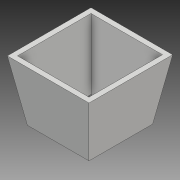
# Autodesk Inventor part: Antenna
Saved by Autodesk Inventor 2017 (Build 210142000, 142)
## iProperties
Created: 2017-01-02
Part Number: Antenna
Material: Generic
Document SubType Name: Modeling
Designer: Sachin Konan
Density: 1 g/cm^3
Appearance: Default
Author: Sachin Konan
Autodesk Inventor part; units mm, degrees
ref_plane "YZ Plane" through (0, 0, 0) normal (1, 0, 0) x (0, 1, 0)
ref_plane "XZ Plane" through (0, 0, 0) normal (0, 1, 0) x (-1, 0, 0)
sketch "Sketch1" plane through (0, 0, 0) normal (0, 0, 1) x (1, 0, 0)
  line L0 (0, 0) -> (49.5, 0)
  line L1 (49.5, 0) -> (49.5, 51.5)
  line L2 (49.5, 51.5) -> (0, 51.5)
  line L3 (0, 51.5) -> (0, 0)
  line L4 (0, 51.5) -> (-6, 51.5)
  line L5 (-6, 51.5) -> (-6, 57.5)
  line L6 (49.5, 0) -> (55.5, 0)
  line L7 (55.5, 0) -> (55.5, -6)
  line L8 (-6, 57.5) -> (55.5, 57.5)
  line L9 (55.5, 57.5) -> (55.5, -6)
  line L10 (55.5, -6) -> (-6, -6)
  line L11 (-6, -6) -> (-6, 57.5)
  dimension "d0" = 49.5
  dimension "d1" = 51.5
  dimension "d2" = 6
  dimension "d3" = 6
  dimension "d4" = 6
  dimension "d5" = 6
  constraints: 24 end point, 4 horizontal, 4 parallel, 4 perpendicular
  measures "d0" distance of L1.end L2.end
  measures "d1" distance of L0.end L1.end
  measures "d2" distance of L2.end L4.end
  measures "d3" distance of L4.end L5.end
  measures "d4" distance of L0.end L6.end
  measures "d5" distance of L6.end L7.end
ref_plane "Work Plane1" through (0, 0, 60) normal (0, 0, 1) x (1, 0, 0)
sketch "Sketch2" plane through (0, 0, 60) normal (0, 0, 1) x (1, 0, 0)
  line L0 (-6, 57.5) -> (55.5, 57.5) projected
  line L1 (-6, -6) -> (-6, 57.5) projected
  line L2 (55.5, -6) -> (-6, -6) projected
  line L3 (55.5, 0) -> (55.5, -6) projected
  line L4 (55.5, 57.5) -> (55.5, -6) projected
  line L5 (-6, 57.5) -> (-16, 57.5)
  line L6 (-16, 57.5) -> (-16, 67.5)
  line L7 (55.5, -6) -> (55.5, -16)
  line L8 (55.5, -16) -> (65.5, -16)
  line L9 (65.5, -16) -> (-16, -16)
  line L10 (-16, -16) -> (-16, 67.5)
  line L11 (-16, 67.5) -> (65.5, 67.5)
  line L12 (65.5, 67.5) -> (65.5, -16)
  point P0 (0, 0)
  point P1 (-6, 51.5)
  dimension "d7" = 10
  dimension "d8" = 10
  dimension "d9" = 10
  dimension "d10" = 10
  constraints: 16 end point, 3 perpendicular, 2 horizontal, 2 parallel, 1 vertical
  measures "d7" distance of L0.start L5.end
  measures "d8" distance of L5.end L6.end
  measures "d9" distance of L2.start L7.end
  measures "d10" distance of L7.end L8.end
loft "Loft1" add profiles "Sketch2", "Sketch1"
shell "Shell1" thickness 5 removed faces 2 at (11.1667, 11.8333, 60) at (14.5, 36.3333, 0)
body "Solid1"
